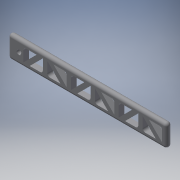
# Autodesk Inventor part: endarm
Saved by Autodesk Inventor 2019 (Build 230136000, 136)
## iProperties
Created: 2019-03-01
Part Number: endarm
Material: Generic
Document SubType Name: Modeling
Designer: s-4036947
Density: 1 g/cm^3
Appearance: Default
Author: s-4036947
Autodesk Inventor part; units mm, degrees
ref_plane "YZ Plane" through (0, 0, 0) normal (1, 0, 0) x (0, 1, 0)
ref_plane "XZ Plane" through (0, 0, 0) normal (0, 1, 0) x (-1, 0, 0)
ref_plane "XY Plane" through (0, 0, 0) normal (0, 0, 1) x (1, 0, 0)
sketch "Sketch1" plane through (0, 0, 0) normal (0, 0, 1) x (1, 0, 0)
  line L0 (14.98, 33.7) -> (197.7852, 33.7)
  line L1 (197.7852, 8.3) -> (14.98, 8.3)
  line L2 (14.98, 8.3) -> (14.98, 33.7)
  arc A0 (30.1177, 21.5547) -> (28.8951, 18.8151) centre (27.68, 21) ccw construction
  line L3 (30.1177, 21.5547) -> (28.8951, 18.8151) construction
  line L4 (-3.175, 42) -> (-122.9515, 42) projected
  line L5 (137.6968, 28.62) -> (137.6968, 13.38)
  line L6 (137.6968, 13.38) -> (122.4568, 28.62)
  line L7 (122.4568, 28.62) -> (137.6968, 28.62)
  line L8 (130.5126, 13.38) -> (115.2726, 28.62)
  line L9 (115.2726, 28.62) -> (115.2726, 13.38)
  line L10 (115.2726, 13.38) -> (130.5126, 13.38)
  line L11 (112.7326, 10.7487) -> (112.7326, 41.4812) construction
  line L12 (87.7684, 28.62) -> (87.7684, 13.38)
  line L13 (87.7684, 13.38) -> (103.0084, 28.62)
  line L14 (103.0084, 28.62) -> (87.7684, 28.62)
  line L15 (94.9526, 13.38) -> (110.1926, 28.62)
  line L16 (110.1926, 28.62) -> (110.1926, 13.38)
  line L17 (110.1926, 13.38) -> (94.9526, 13.38)
  line L18 (85.2284, 8.9371) -> (85.2284, 32.7241) construction
  line L19 (32.76, 28.62) -> (32.76, 13.38)
  line L20 (32.76, 13.38) -> (48, 28.62)
  line L21 (48, 28.62) -> (32.76, 28.62)
  line L22 (39.9442, 13.38) -> (55.1842, 28.62)
  line L23 (55.1842, 28.62) -> (55.1842, 13.38)
  line L24 (55.1842, 13.38) -> (39.9442, 13.38)
  line L25 (82.6884, 28.62) -> (82.6884, 13.38)
  line L26 (82.6884, 13.38) -> (67.4484, 28.62)
  line L27 (67.4484, 28.62) -> (82.6884, 28.62)
  line L28 (75.5042, 13.38) -> (60.2642, 28.62)
  line L29 (60.2642, 13.38) -> (75.5042, 13.38)
  line L30 (60.2642, 28.62) -> (60.2642, 13.38)
  line L31 (140.2368, 33.7) -> (140.2368, 8.3) construction
  line L32 (142.7768, 28.62) -> (142.7768, 13.38)
  line L33 (142.7768, 13.38) -> (158.0168, 28.62)
  line L34 (158.0168, 28.62) -> (142.7768, 28.62)
  line L35 (149.961, 13.38) -> (165.201, 28.62)
  line L36 (165.201, 28.62) -> (165.201, 13.38)
  line L37 (165.201, 13.38) -> (149.961, 13.38)
  line L38 (192.7052, 28.62) -> (192.7052, 13.38)
  line L39 (192.7052, 13.38) -> (177.4652, 28.62)
  line L40 (177.4652, 28.62) -> (192.7052, 28.62)
  line L41 (185.521, 13.38) -> (170.281, 28.62)
  line L42 (170.281, 13.38) -> (185.521, 13.38)
  line L43 (170.281, 28.62) -> (170.281, 13.38)
  line L44 (197.7852, 33.7) -> (197.7852, 8.3)
  arc A1 (30.379, 21.5269) -> (29.0903, 18.6392) centre (27.68, 21) ccw
  line L45 (29.0903, 18.6392) -> (30.379, 21.5269)
  point P0 (0, 0)
  dimension "d0" = 12.7
  dimension "d1" = 12.7
  dimension "d2" = 12.7
  dimension "d7" = 45
  dimension "d9" = 5.08
  dimension "d10" = 5.08
  dimension "d11" = 5.08
  dimension "d12" = 0
  dimension "d14" = 2.54
  dimension "d15" = 2.54
  dimension "d16" = 5.08
  dimension "d23" = 2.54
  dimension "d24" = 5.08
  dimension "d29" = 5.5
  dimension "d30" = 2.5
  dimension "d31" = 0.25
  constraints: 90 end point, 35 symmetric about line, 8 point on line, 6 parallel, 5 vertical, 2 perpendicular, 2 point on circle, 1 centre point, 1 coincident, 1 horizontal
  measures "d0" distance from line of L0 A0.centre
  measures "d1" distance from line of L1 A0.centre
  measures "d2" distance from line of L2 A0.centre
  measures "d7" angle of L6 L5
  measures "d9" distance between parallel lines of L0 L7
  measures "d10" distance from line of L1 L5.end
  measures "d11" distance between parallel lines of L8 L6
  measures "d12" distance from line of L10 L5.end
  measures "d14" distance between parallel lines of L11 L9
  measures "d15" distance between parallel lines of L18 L12
  measures "d16" distance from line of A0.centre L19
  measures "d23" distance between parallel lines of L31 L5
  measures "d24" distance between parallel lines of L44 L38
  measures "d29" diameter of A1
  measures "d30" radius of A0
  measures "d31" distance between parallel lines of L45 L3
extrude "Extrusion4" add sketch "Sketch1" along normal blind 6.35
fillet "Fillet7" radius 3.175 12 edges at (106.3826, 8.3, 6.35) (106.3826, 8.3, 0) (106.3826, 33.7, 0) (106.3826, 33.7, 6.35) (197.7852, 21, 6.35) (197.7852, 21, 0) (197.7852, 33.7, 3.175) (197.7852, 8.3, 3.175) (14.98, 21, 6.35) (14.98, 21, 0) (14.98, 8.3, 3.175) (14.98, 33.7, 3.175)
fillet "Fillet8" radius 3.175 12 edges at (55.1842, 13.38, 3.175) (60.2642, 13.38, 3.175) (32.76, 28.62, 3.175) (82.6884, 28.62, 3.175) (87.7684, 28.62, 3.175) (110.1926, 13.38, 3.175) (115.2726, 13.38, 3.175) (137.6968, 28.62, 3.175) (142.7768, 28.62, 3.175) (165.201, 13.38, 3.175) (170.281, 13.38, 3.175) (192.7052, 28.62, 3.175)
equation "\"d1\" = d0"
equation "\"d24\" = d9"
body "Solid4"
